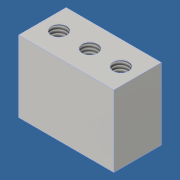
# Autodesk Inventor part: Alu_Belt_tens
Saved by Autodesk Inventor 2016 (Build 200138000, 138)
## iProperties
Created: 2015-09-19
Part Number: Alu_Belt_tens
Material: Aluminium 6061
Document SubType Name: Modeling
Designer: 4ndreas
Density: 2.7 g/cm^3
Appearance: Aluminium - flach
Mass: 7.09702 g
Surface Area: 17.088 cm^2
Volume: 2.62853 cm^3
Author: 4ndreas
Autodesk Inventor part; units mm, degrees
ref_plane "YZ Plane" through (0, 0, 0) normal (1, 0, 0) x (0, 1, 0)
ref_plane "XZ Plane" through (0, 0, 0) normal (0, 1, 0) x (-1, 0, 0)
ref_plane "XY Plane" through (0, 0, 0) normal (0, 0, 1) x (1, 0, 0)
sketch "Skizze1" plane through (0, 0, 0) normal (0, 0, 1) x (1, 0, 0)
  line L0 (-10, -5) -> (10, -5)
  line L1 (10, -5) -> (10, 5)
  line L2 (10, 5) -> (-10, 5)
  line L3 (-10, 5) -> (-10, -5)
  line L4 (-10, -5) -> (10, 5) construction
  line L5 (10, -5) -> (-10, 5) construction
  circle A0 centre (0, 0) radius 2
  circle A1 centre (-6.5, 0) radius 2
  circle A2 centre (6.5, 0) radius 2
  line L6 (-10, 0) -> (10, 0) construction
  dimension "d0" = 10
  dimension "d1" = 20
  dimension "d2" = 4
  dimension "d3" = 6.5
  dimension "d4" = 6.5
  constraints: 14 end point, 4 midpoint, 3 centre point, 2 equal radius, 2 parallel, 2 point on line, 1 coincident, 1 horizontal, 1 perpendicular
  measures "d0" distance between parallel lines of L0 L2
  measures "d1" distance between parallel lines of L1 L3
  measures "d2" diameter of A0
  measures "d3" distance of point (0, 0) A1.centre
  measures "d4" distance of point (0, 0) A2.centre
extrude "Extrusion1" add sketch "Skizze1" along normal blind 15 contours L3 L2 L1 L0 | A0 | A1 | A2
sketch "Skizze2" plane through (0, 0, 15) normal (0, 0, 1) x (1, 0, 0)
  point P0 (0, 0)
hole "Bohrung1" at (0, 0, 15) direction (0, 0, -1) diameter 3.242 end through all thread size "M4x0.7" class "6H" standard "ANSI Metric M Profile"
sketch "Skizze3" plane through (0, 0, 0) normal (0, 0, -1) x (-1, 0, 0)
  point P0 (0, 0)
  point P1 (-6.5, 0)
  point P2 (6.5, 0)
hole "Bohrung2" at (6.5, 0, 0) at (-6.5, 0, 0) direction (0, 0, 1) diameter 3.242 end through all thread size "M4x0.7" class "6H" standard "ANSI Metric M Profile"
equation "\"d4\" = d3"
